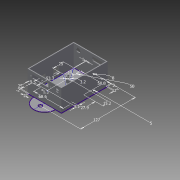
# Autodesk Inventor part: LED pump controller
Saved by Autodesk Inventor 2013 SP2 (Build 170200200, 200)
## iProperties
Created: 2013-04-19
Part Number: LED pump controller
Material: Generic
Document SubType Name: Modeling
Designer: kthorn
Density: 1 g/cm^3
Author: kthorn
Autodesk Inventor part; units mm, degrees
ref_plane "YZ Plane" through (0, 0, 0) normal (1, 0, 0) x (0, 1, 0)
ref_plane "XZ Plane" through (0, 0, 0) normal (0, 1, 0) x (-1, 0, 0)
ref_plane "XY Plane" through (0, 0, 0) normal (0, 0, 1) x (1, 0, 0)
sketch "Sketch1" plane through (0, 0, 0) normal (0, 0, 1) x (1, 0, 0)
  line L0 (-35.3, 51.65) -> (39.3, 51.65)
  line L1 (39.3, 51.65) -> (39.3, -51.65)
  line L2 (39.3, -51.65) -> (-35.3, -51.65)
  line L3 (-35.3, -51.65) -> (-35.3, 51.65)
  line L4 (-35.3, 51.65) -> (39.3, -51.65) construction
  line L5 (39.3, 51.65) -> (-35.3, -51.65) construction
  line L6 (34.3, 26.65) -> (-34.3, 26.65) construction
  line L7 (-34.3, 26.65) -> (-34.3, -26.65) construction
  line L8 (-34.3, -26.65) -> (34.3, -26.65) construction
  line L9 (34.3, -26.65) -> (34.3, 26.65) construction
  line L10 (34.3, 26.65) -> (-34.3, -26.65) construction
  line L11 (-34.3, 26.65) -> (34.3, -26.65) construction
  circle A0 centre (-20.3, 24.05) radius 1.6 construction
  circle A1 centre (-21.6, -24.15) radius 1.6 construction
  circle A2 centre (30.5, 8.85) radius 1.6 construction
  circle A3 centre (30.5, -19.05) radius 1.6 construction
  line L12 (-37.3, 53.65) -> (41.3, 53.65)
  line L13 (41.3, 53.65) -> (41.3, -53.65)
  line L14 (41.3, -53.65) -> (-37.3, -53.65)
  line L15 (-37.3, -53.65) -> (-37.3, 53.65)
  line L16 (-37.3, 53.65) -> (41.3, -53.65) construction
  line L17 (41.3, 53.65) -> (-37.3, -53.65) construction
  line L18 (30.5, 53.65) -> (30.5, -53.65) construction
  arc A4 (27, 53.65) -> (-23, 53.65) centre (2, 53.65) ccw
  arc A5 (-23, -53.65) -> (27, -53.65) centre (2, -53.65) ccw
  circle A6 centre (2, 63.5) radius 4
  circle A7 centre (2, -63.5) radius 4
  line L19 (2, -63.5) -> (2, 63.5) construction
  line L20 (2, 78.65) -> (2, 63.5) construction
  line L21 (2, -63.5) -> (2, -78.65) construction
  point P0 (0, 0)
  dimension "d0" = 53.3
  dimension "d2" = 68.6
  dimension "d3" = 14
  dimension "d4" = 2.5
  dimension "d5" = 50.8
  dimension "d6" = 27.9
  dimension "d7" = 5.1
  dimension "d8" = 3.2
  dimension "d9" = 25
  dimension "d10" = 1
  dimension "d11" = 2
  dimension "d12" = 2
  dimension "d59" = 5
  dimension "d62" = 25
  dimension "d63" = 2
  dimension "d64" = 2
  dimension "d92" = 15.2
  dimension "d94" = 1.3
  dimension "d95" = 50
  dimension "d96" = 8
  dimension "d99" = 127
  constraints: 44 end point, 8 centre point, 8 point on line, 6 parallel, 6 point on circle, 5 equal radius, 5 perpendicular, 4 midpoint, 3 horizontal, 2 collinear
  measures "d0" distance of L6.end L7.end
  measures "d2" distance of L7.end L8.end
  measures "d3" distance from line of L7 A0.centre
  measures "d4" distance from line of L8 A1.centre
  measures "d5" horizontal distance of A2.centre A0.centre
  measures "d6" distance of A3.centre A2.centre
  measures "d7" vertical distance of A3.centre A1.centre
  measures "d8" diameter of A0
  measures "d9" distance between parallel lines of L0 L6
  measures "d10" distance between parallel lines of L3 L7
  measures "d11" distance between parallel lines of L12 L0
  measures "d12" distance between parallel lines of L13 L1
  measures "d59" distance between parallel lines of L1 L9
  measures "d62" distance between parallel lines of L2 L8
  measures "d63" distance between parallel lines of L14 L2
  measures "d64" distance between parallel lines of L15 L3
  measures "d92" vertical distance of A2.centre A0.centre
  measures "d94" horizontal distance of A1.centre A0.centre
  measures "d95" diameter of A4
  measures "d96" diameter of A6
  measures "d99" distance of L19.start L19.end
extrude "Extrusion1" add sketch "Sketch1" against normal blind 2 contours L0 L1 L2 L3 | L12 L13 L14 L15
extrude "Extrusion2" add sketch "Sketch1" along normal blind 50 contours L12 L13 L14 L15
sketch "Sketch2" plane through (0, 0, 0) normal (0, 0, 1) x (1, 0, 0)
  circle A0 centre (-21.6, -24.15) radius 1.6 construction
  circle A1 centre (-20.3, 24.05) radius 4.15
  circle A2 centre (-21.6, -24.15) radius 4.15
  circle A3 centre (30.5, -19.05) radius 4.15
  circle A4 centre (30.5, 8.85) radius 4.15
  circle A5 centre (-20.3, 24.05) radius 2.15
  circle A6 centre (30.5, 8.85) radius 2.15
  circle A7 centre (-21.6, -24.15) radius 2.15
  circle A8 centre (30.5, -19.05) radius 2.15
  point P0 (0, 0)
  dimension "d17" = 8.3
  dimension "d19" = 4.3
  constraints: 8 centre point, 8 coincident, 6 equal radius
  measures "d17" diameter of A1
  measures "d19" diameter of A5
extrude "Extrusion3" add sketch "Sketch2" along normal blind 5
sketch "Sketch6" plane through (-37.3, 53.65, -2) normal (0, 1, 0) x (1, 0, 0)
  line L0 (78.6, -52) -> (78.6, 0) projected
  line L1 (0, 0) -> (0, -52) projected
  line L2 (0, -42) -> (78.6, -42) construction
  arc A0 (9.2389, -38.11) -> (15.3611, -38.11) centre (12.3, -42) ccw
  line L3 (78.6, -52) -> (0, -52) projected
  line L4 (12.3, -42) -> (12.3, -38.11) construction
  line L5 (9.2389, -38.11) -> (15.3611, -38.11)
  line L6 (68.6, -46.3) -> (68.6, -39.95)
  line L7 (66.35, -37.7) -> (47.25, -37.7)
  line L8 (45, -39.95) -> (45, -46.3)
  line L9 (45, -46.3) -> (68.6, -46.3)
  line L10 (47.25, -37.7) -> (45, -39.95)
  line L11 (68.6, -39.95) -> (66.35, -37.7)
  line L12 (68.6, -46.3) -> (68.6, -41.3) construction
  line L13 (56.8, -37.7) -> (56.8, -46.3) construction
  point P0 (37.3, -2)
  point P1 (45, -37.7)
  point P2 (68.6, -37.7)
  point P3 (56.8, -42)
  dimension "d46" = 9.9
  dimension "d54" = 12.3
  dimension "d65" = 3.89
  dimension "d122" = 23.6
  dimension "d123" = 8.6
  dimension "d124" = 2.25
  dimension "d125" = 2.25
  dimension "d126" = 2.25
  dimension "d127" = 2.25
  dimension "d128" = 5
  dimension "d129" = 10
  dimension "d130" = 10
  constraints: 22 end point, 8 point on line, 4 midpoint, 4 perpendicular, 2 parallel, 2 point on circle, 1 centre point
  measures "d46" diameter of A0
  measures "d54" distance from line of L1 L4.start
  measures "d65" distance of L4.start L4.end
  measures "d122" distance of L8.end L6.start
  measures "d123" distance of point (45, -37.7) L8.end
  measures "d124" distance of L10.start point (45, -37.7)
  measures "d125" distance of L8.start point (45, -37.7)
  measures "d126" distance of L6.end point (68.6, -37.7)
  measures "d127" distance of L7.start point (68.6, -37.7)
  measures "d128" distance of L6.start L12.end
  measures "d129" distance between parallel lines of L0 L6
  measures "d130" distance between parallel lines of L3 L2
extrude "Extrusion6" cut sketch "Sketch6" against normal up to next
sketch "Sketch7" plane through (0, 0, 0) normal (0, 0, 1) x (1, 0, 0)
  circle A0 centre (30.5, -19.05) radius 4.15 projected
  circle A1 centre (30.5, 8.85) radius 4.15 projected
  line L0 (-14.3, -17.05) -> (24.5, -17.05)
  line L1 (24.5, -17.05) -> (24.5, -21.05)
  line L2 (24.5, -21.05) -> (-14.3, -21.05)
  line L3 (-14.3, -21.05) -> (-14.3, -17.05)
  line L4 (-34.3, -26.65) -> (34.3, -26.65) construction
  line L5 (34.3, 26.65) -> (-34.3, 26.65) construction
  line L6 (34.3, -26.65) -> (34.3, 26.65) construction
  line L7 (-34.3, 26.65) -> (-34.3, -26.65) construction
  line L8 (24.5, 16.65) -> (-14.3, 16.65)
  line L9 (-14.3, 16.65) -> (-14.3, 12.65)
  line L10 (-14.3, 12.65) -> (24.5, 12.65)
  line L11 (24.5, 12.65) -> (24.5, 16.65)
  point P0 (0, 0)
  point P1 (24.5, -19.05)
  dimension "d79" = 4
  dimension "d80" = 20
  dimension "d81" = 6
  dimension "d82" = 6
  dimension "d83" = 20
  dimension "d86" = 10
  dimension "d87" = 0
  constraints: 16 end point, 4 parallel, 2 horizontal, 2 perpendicular, 1 collinear, 1 midpoint
  measures "d79" distance of L2.end L0.start
  measures "d80" distance between parallel lines of L7 L3
  measures "d81" distance from line of L1 A0.centre
  measures "d82" distance from line of L11 A1.centre
  measures "d83" distance between parallel lines of L7 L9
  measures "d86" distance between parallel lines of L5 L8
  measures "d87" vertical distance of A0.centre point (24.5, -19.05)
extrude "Extrusion7" add sketch "Sketch7" along normal blind 8 contours L0 L1 L2 L3 | L11 L10 L9 L8
sketch "Sketch4" plane through (-37.3, -53.65, -2) normal (-1, 0, 0) x (0, 0, 1)
  line L0 (11.5, 71.3) -> (23.5, 71.3)
  line L1 (23.5, 71.3) -> (23.5, 58.3)
  line L2 (23.5, 58.3) -> (11.5, 58.3)
  line L3 (11.5, 58.3) -> (11.5, 71.3)
  line L4 (11.5, 71.3) -> (23.5, 58.3) construction
  line L5 (23.5, 71.3) -> (11.5, 58.3) construction
  line L6 (23.5, 30.25) -> (11.5, 30.25)
  line L7 (11.5, 30.25) -> (11.5, 40.25)
  line L8 (11.5, 40.25) -> (23.5, 40.25)
  line L9 (23.5, 40.25) -> (23.5, 30.25)
  line L10 (23.5, 30.25) -> (11.5, 40.25) construction
  line L11 (11.5, 30.25) -> (23.5, 40.25) construction
  line L12 (2, 0) -> (2, 107.3) projected
  line L13 (7, 73.55) -> (7, 81.85) projected
  line L14 (10, 36.6) -> (10, 32.6) projected
  line L15 (0, 107.3) -> (52, 107.3) projected
  line L16 (0, 0) -> (0, 107.3) projected
  line L17 (52, 0) -> (0, 0) projected
  line L18 (52, 107.3) -> (52, 0) projected
  point P0 (2, 53.65)
  point P1 (2, 80.3)
  point P2 (2, 80.3)
  point P3 (2, 80.3)
  point P4 (2, 27)
  point P5 (2, 27)
  point P6 (2, 27)
  point P7 (17.5, 64.8)
  point P8 (17.5, 35.25)
  point P9 (2, 0)
  dimension "d22" = 13
  dimension "d24" = 12
  dimension "d26" = 9
  dimension "d27" = 12
  dimension "d28" = 10
  dimension "d31" = 3.25
  dimension "d88" = 1.5
  dimension "d90" = 1.5
  constraints: 24 end point, 4 midpoint, 4 parallel, 2 horizontal, 2 perpendicular, 1 other
  measures "d22" distance of L0.end L1.end
  measures "d24" distance of L0.start L0.end
  measures "d26" distance from line of point (2, 80.3) L0
  measures "d27" distance of L7.end L8.end
  measures "d28" distance of L8.end L6.start
  measures "d31" distance from line of point (2, 27) L6
  measures "d88" distance between parallel lines of L7 L14
  measures "d90" distance between parallel lines of L3 L14
extrude "Extrusion4" cut sketch "Sketch4" against normal up to surface (2 mm away) contours L0 L1 L2 L3 | L6 L7 L8 L9
extrude "Extrusion8" add sketch "Sketch1" against normal up to surface (2 mm away) contours A4 L12 | L14 A5
sketch "Sketch8" plane through (-37.3, -53.65, 50) normal (0, -1, 0) x (1, 0, 0)
  line L0 (78.6, 0) -> (78.6, -52) projected
  line L1 (0, 0) -> (78.6, 0) projected
  line L2 (0, 0) -> (0, -52) projected
  line L3 (11.5, -5.85) -> (48.5, -5.85)
  line L4 (48.5, -5.85) -> (48.5, -14.15)
  line L5 (48.5, -14.15) -> (11.5, -14.15)
  line L6 (11.5, -14.15) -> (11.5, -5.85)
  line L7 (48.5, -10) -> (52.5, -10) construction
  line L8 (11.5, -10) -> (7.5, -10) construction
  circle A0 centre (7.5, -10) radius 1.5
  circle A1 centre (52.5, -10) radius 1.5
  line L9 (0, -10) -> (7.5, -10) construction
  line L10 (7.5, -10) -> (7.5, 0) construction
  circle A2 centre (68.6, -10) radius 4.05
  line L11 (68.6, -10) -> (68.6, 0) construction
  line L12 (68.6, -10) -> (78.6, -10) construction
  point P0 (37.3, -50)
  dimension "d100" = 8.3
  dimension "d102" = 37
  dimension "d103" = 4
  dimension "d104" = 3
  dimension "d105" = 10
  dimension "d106" = 7.5
  dimension "d107" = 8.1
  dimension "d108" = 10
  constraints: 20 end point, 5 perpendicular, 4 point on line, 3 centre point, 2 coincident, 2 collinear, 2 equal length, 2 midpoint, 2 parallel, 1 equal radius, 1 horizontal
  measures "d100" distance of L3.end L4.end
  measures "d102" distance of L3.start L3.end
  measures "d103" distance of L8.end L8.start
  measures "d104" diameter of A0
  measures "d105" distance of L8.end L10.end
  measures "d106" distance of L9.start L8.end
  measures "d107" diameter of A2
  measures "d108" distance of L11.start L12.end
extrude "Extrusion9" cut sketch "Sketch8" against normal up to next
equation "\"d125\" = d124"
equation "\"d126\" = d124"
equation "\"d127\" = d126"
body "Solid1"
